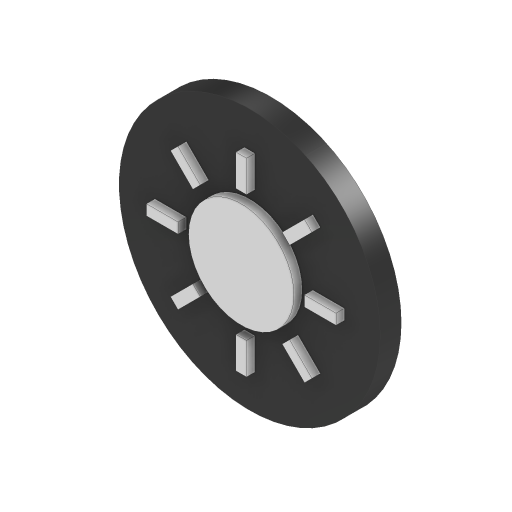
# Autodesk Inventor part: button_plate_brightness
Saved by Autodesk Inventor 2023 (Build 270158000, 158)
## iProperties
Created: 2025-02-19
Part Number: button_plate_brightness
Material: Všeobecné
Document SubType Name: Modeling
Designer: Marek
Density: 1 g/cm^3
Appearance: Výchozí
Author: Marek
Autodesk Inventor part; units mm, degrees
ref_plane "YZ Plane" through (0, 0, 0) normal (1, 0, 0) x (0, 1, 0)
ref_plane "XZ Plane" through (0, 0, 0) normal (0, 1, 0) x (-1, 0, 0)
ref_plane "XY Plane" through (0, 0, 0) normal (0, 0, 1) x (1, 0, 0)
sketch "Náčrt1" plane through (0, 0, 0) normal (0, 0, 1) x (1, 0, 0)
  line L0 (0, 8.68) -> (0, -8.68) projected
  line L1 (-8.68, 0) -> (8.68, 0) projected
  circle A0 centre (0, 0) radius 6.2
  dimension "d0" = 12.4
  constraints: 1 centre point, 1 coincident
  measures "d0" diameter of A0
extrude "Vysunutí1" add sketch "Náčrt1" along normal blind 1
sketch "Náčrt2" plane through (0, 0, 1) normal (0, 0, 1) x (1, 0, 0)
  line L0 (-8.68, 0) -> (8.68, 0) projected
  line L1 (0, 8.68) -> (0, -8.68) projected
  circle A0 centre (0, 0) radius 2.5
  line L2 (-0.25, 3) -> (0.25, 3)
  line L3 (0.25, 3) -> (0.25, 4.5)
  line L4 (0.25, 4.5) -> (-0.25, 4.5)
  line L5 (-0.25, 4.5) -> (-0.25, 3)
  line L6 (-2.2981, 1.9445) -> (-1.9445, 2.2981)
  line L7 (-1.9445, 2.2981) -> (-3.0052, 3.3588)
  line L8 (-3.0052, 3.3588) -> (-3.3588, 3.0052)
  line L9 (-3.3588, 3.0052) -> (-2.2981, 1.9445)
  line L10 (-3, -0.25) -> (-3, 0.25)
  line L11 (-3, 0.25) -> (-4.5, 0.25)
  line L12 (-4.5, 0.25) -> (-4.5, -0.25)
  line L13 (-4.5, -0.25) -> (-3, -0.25)
  line L14 (-1.9445, -2.2981) -> (-2.2981, -1.9445)
  line L15 (-2.2981, -1.9445) -> (-3.3588, -3.0052)
  line L16 (-3.3588, -3.0052) -> (-3.0052, -3.3588)
  line L17 (-3.0052, -3.3588) -> (-1.9445, -2.2981)
  line L18 (0.25, -3) -> (-0.25, -3)
  line L19 (-0.25, -3) -> (-0.25, -4.5)
  line L20 (-0.25, -4.5) -> (0.25, -4.5)
  line L21 (0.25, -4.5) -> (0.25, -3)
  line L22 (2.2981, -1.9445) -> (1.9445, -2.2981)
  line L23 (1.9445, -2.2981) -> (3.0052, -3.3588)
  line L24 (3.0052, -3.3588) -> (3.3588, -3.0052)
  line L25 (3.3588, -3.0052) -> (2.2981, -1.9445)
  line L26 (3, 0.25) -> (3, -0.25)
  line L27 (3, -0.25) -> (4.5, -0.25)
  line L28 (4.5, -0.25) -> (4.5, 0.25)
  line L29 (4.5, 0.25) -> (3, 0.25)
  line L30 (1.9445, 2.2981) -> (2.2981, 1.9445)
  line L31 (2.2981, 1.9445) -> (3.3588, 3.0052)
  line L32 (3.3588, 3.0052) -> (3.0052, 3.3588)
  line L33 (3.0052, 3.3588) -> (1.9445, 2.2981)
  dimension "d3" = 5
  dimension "d4" = 0.5
  dimension "d5" = 1.5
  dimension "d6" = 3
  dimension "d9" = 360
  constraints: 64 end point, 2 parallel, 1 centre point, 1 coincident, 1 horizontal, 1 perpendicular, 66 other
  measures "d3" diameter of A0
  measures "d4" distance between parallel lines of L5 L3
  measures "d5" distance between parallel lines of L2 L4
  measures "d6" distance between parallel lines of L2 L0
extrude "Vysunutí2" add sketch "Náčrt2" along normal blind 0.4
